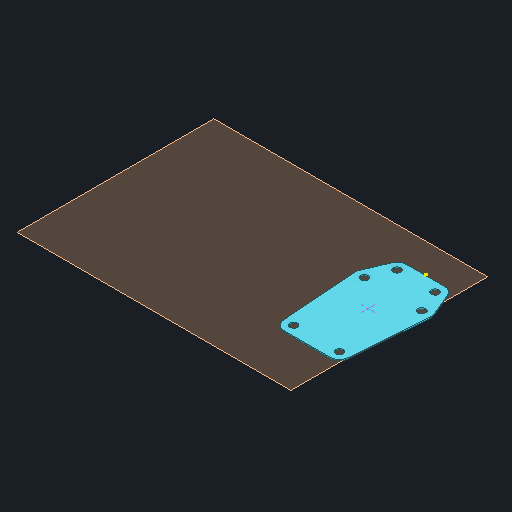
# Autodesk Inventor part: body_composition
Saved by Autodesk Inventor 2026 (Build 300175000, 175)
## iProperties
Created: 2026-04-26
Part Number: body_composition
Material: Сталь
Document SubType Name: Modeling
Designer: user
Density: 7.85 g/cm^3
Appearance: Серо-синий
Mass: 1256.55 g
Surface Area: 1105.69 cm^2
Volume: 160.07 cm^3
Author: user
Autodesk Inventor part; units mm, degrees
ref_plane "YZ Plane" through (0, 0, 0) normal (1, 0, 0) x (0, 1, 0)
ref_plane "XY Plane" through (0, 0, 0) normal (0, 0, 1) x (1, 0, 0)
ref_plane "РабПлоскость1" through (0, 500, 0) normal (0, 1, 0) x (-1, 0, 0)
sketch "Эскиз5" plane through (0, 500, 0) normal (0, 1, 0) x (-1, 0, 0)
  circle A0 centre (-50, 25) radius 10
  line L0 (0, -2.2566) -> (0, 604.845)
  circle A1 centre (-75, 85) radius 10
  circle A2 centre (-60, 285) radius 10
  arc A3 (-60, 310) -> (-84.93, 286.8697) centre (-60, 285) ccw
  arc A4 (-99.93, 86.8697) -> (-98.0769, 75.3846) centre (-75, 85) ccw
  arc A5 (-73.0769, 15.3846) -> (-50, 0) centre (-50, 25) ccw
  line L1 (-84.93, 286.8697) -> (-99.93, 86.8697)
  line L2 (-98.0769, 75.3846) -> (-73.0769, 15.3846)
  line L3 (-60, 310) -> (0, 310)
  line L4 (-50, 0) -> (0, 0)
  line L5 (98.0769, 75.3846) -> (73.0769, 15.3846)
  arc A6 (98.0769, 75.3846) -> (99.93, 86.8697) centre (75, 85) ccw
  circle A7 centre (75, 85) radius 10
  arc A8 (50, 0) -> (73.0769, 15.3846) centre (50, 25) ccw
  circle A9 centre (50, 25) radius 10
  line L6 (50, 0) -> (0, 0)
  line L7 (84.93, 286.8697) -> (99.93, 86.8697)
  circle A10 centre (60, 285) radius 10
  arc A11 (84.93, 286.8697) -> (60, 310) centre (60, 285) ccw
  line L8 (60, 310) -> (0, 310)
  dimension "d19" = 100
  dimension "d20" = 150
  dimension "d21" = 120
  dimension "d22" = 200
  dimension "d23" = 60
  dimension "d24" = 20
  dimension "d25" = 50
  constraints: 18 end point, 12 centre point, 12 point on circle, 12 symmetric about line, 7 coincident, 6 tangent, 4 equal radius, 2 perpendicular, 2 point on line, 1 vertical, 6 other
  measures "d19" diameter of A0.centre L0
  measures "d20" diameter of A1.centre L0
  measures "d21" diameter of A2.centre L0
  measures "d22" vertical distance of A1.centre A2.centre
  measures "d23" vertical distance of A1.centre A0.centre
  measures "d24" diameter of A0
  measures "d25" diameter of A3
extrude "Выдавливание5" add sketch "Эскиз5" along normal blind 3
sketch "Эскиз7" plane through (0, 503, 0) normal (0, 1, 0) x (1, 0, 0)
  point P0 (0, 0)
  point P1 (0, -149.6314)
equation "\"d19\" = d26"
equation "\"d20\" = d27"
equation "\"d21\" = d28"
equation "\"d22\" = d29"
equation "\"d23\" = d30"
equation "\"d24\" = d31"
equation "\"d32\" = thickness_steel"
equation "\"tolerance_plazma\" = 0.1"
equation "\"thickness_steel\" = 3"
equation "\"d_main_screw_holes\" = 6.1"
equation "\"d_main_shaft\" = 16"
equation "\"thickness_profile_tibea\" = 4"
equation "\"thickness_profile_femur\" = 3"
equation "\"width_shaft_shift\" = 35"
equation "\"width_flattened_surface\" = 12"
equation "\"d26\" = 100"
equation "\"d27\" = 150"
equation "\"d28\" = 120"
equation "\"d29\" = 200"
equation "\"d30\" = 60"
equation "\"d31\" = 20"
